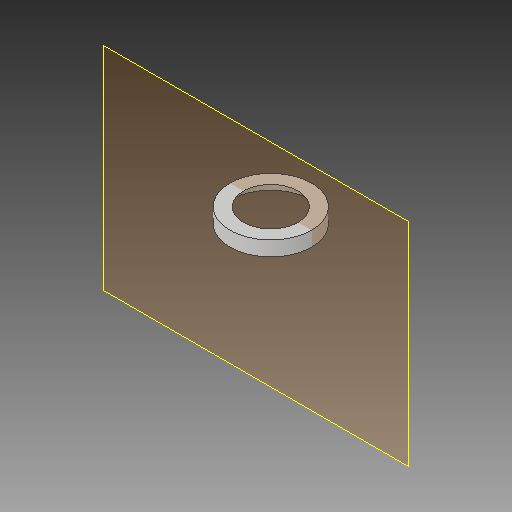
# Autodesk Inventor part: Part2
Saved by Autodesk Inventor 2019 (Build 230136000, 136)
## iProperties
Created: 2018-12-15
Part Number: Part2
Material: Generic
Document SubType Name: Modeling
Designer: assman
Density: 1 g/cm^3
Appearance: Default
Author: assman
Autodesk Inventor part; units mm, degrees
ref_plane "YZ Plane" through (0, 0, 0) normal (1, 0, 0) x (0, 1, 0)
ref_plane "XZ Plane" through (0, 0, 0) normal (0, 1, 0) x (-1, 0, 0)
ref_plane "XY Plane" through (0, 0, 0) normal (0, 0, 1) x (1, 0, 0)
ref_plane "Work Plane1" through (0, 285.3175, 0) normal (0, 0, 1) x (-1, 0, 0)
sketch "Sketch1" plane through (0, 285.3175, 0) normal (0, 0, 1) x (-1, 0, 0)
  line L0 (92, -45.3253) -> (32, -45.3253) projected
  line L1 (32, -34.5335) -> (42, -45.3253)
  line L2 (32, -45.3253) -> (42, -45.3253)
  line L3 (42, -45.3253) -> (32, -34.5335)
  line L4 (32, -34.5335) -> (32, -45.3253)
  line L5 (62, -0.0782) -> (62, -47.9486) construction
  point P0 (0, 285.3175)
  constraints: 10 end point, 2 perpendicular, 1 collinear, 3 other
revolve "Revolution1" add sketch "Sketch1" angle 360 about axis through (-62, 285.3957, 0) along (0, 1, 0)
body "Solid1"
